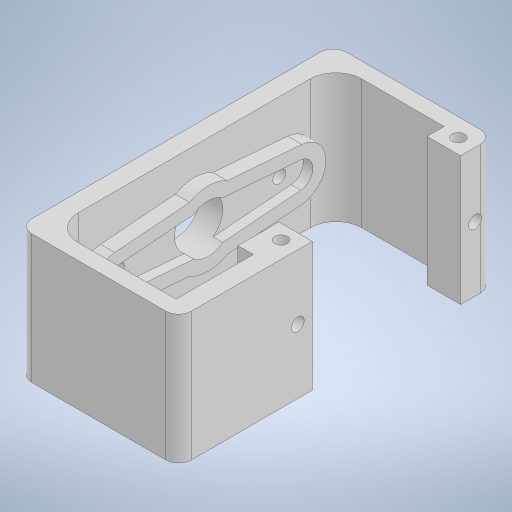
# Autodesk Inventor part: joint4
Saved by Autodesk Inventor 2023 (Build 270158000, 158)
## iProperties
Created: 2023-04-30
Part Number: joint4
Material: 一般
Document SubType Name: Modeling
Designer: taka2
Density: 1 g/cm^3
Appearance: 既定
Author: taka2
Autodesk Inventor part; units mm, degrees
ref_plane "YZ Plane" through (0, 0, 0) normal (1, 0, 0) x (0, 1, 0)
ref_plane "XZ Plane" through (0, 0, 0) normal (0, 1, 0) x (-1, 0, 0)
ref_plane "XY Plane" through (0, 0, 0) normal (0, 0, 1) x (1, 0, 0)
sketch "スケッチ1" plane through (0, 0, 0) normal (0, 1, 0) x (-1, 0, 0)
  line L0 (34.0614, 0) -> (-44.6235, 0)
  line L1 (0, 24.4) -> (0, -24.4)
  line L2 (0, -24.4) -> (-24.8, -24.4)
  line L3 (-24.8, -24.4) -> (-24.8, -22)
  line L4 (-24.8, -22) -> (-2.8, -22)
  line L5 (-2.8, -22) -> (-2.8, 22)
  line L6 (-2.8, 22) -> (-24.8, 22)
  line L7 (-24.8, 22) -> (-24.8, 24.4)
  line L8 (-24.8, 24.4) -> (0, 24.4)
  point P0 (0, 0)
  dimension "d0" = 2.8
  dimension "d1" = 48.8
  dimension "d2" = 24.4
  dimension "d3" = 2.4
  dimension "d4" = 2.4
  dimension "d5" = 22
  constraints: 18 end point, 4 perpendicular, 3 horizontal, 2 vertical, 1 collinear, 1 midpoint, 1 point on line
  measures "d0" distance between parallel lines of L1 L5
  measures "d1" distance of L1.start L1.end
  measures "d2" distance of L1.start point (0, 0)
  measures "d3" distance between parallel lines of L8 L6
  measures "d4" distance between parallel lines of L4 L2
  measures "d5" distance of L3.end L4.end
extrude "押し出し1" add sketch "スケッチ1" along normal blind 20
sketch "スケッチ2" plane through (2.8, 0, 22) normal (1, 0, 0) x (0, 0, -1)
  line L0 (0, 20) -> (44, 20) projected
  line L1 (22, 20) -> (22, 0)
  line L2 (0, 0) -> (44, 0) projected
  line L3 (-2.4, 0) -> (-2.4, 20) projected
  line L4 (-2.4, 10) -> (46.4, 10)
  line L5 (46.4, 0) -> (46.4, 20) projected
  circle A0 centre (22, 10) radius 3.75
  arc A1 (7.6386, 12.0436) -> (7.6386, 7.9564) centre (7.8, 10) ccw
  line L6 (19.75, 13) -> (7.6386, 12.0436)
  line L7 (19.75, 7) -> (7.6386, 7.9564)
  circle A2 centre (9.5, 10) radius 1
  arc A3 (36.3614, 7.9564) -> (36.3614, 12.0436) centre (36.2, 10) ccw
  line L8 (24.25, 13) -> (36.3614, 12.0436)
  line L9 (24.25, 7) -> (36.3614, 7.9564)
  circle A4 centre (34.5, 10) radius 1
  line L10 (19.0799, 14.9533) -> (7.4812, 14.0374)
  arc A5 (7.4812, 14.0374) -> (7.4812, 5.9626) centre (7.8, 10) ccw
  line L11 (7.4812, 5.9626) -> (19.0799, 5.0467)
  circle A6 centre (22, 10) radius 5.75
  line L12 (24.9201, 14.9533) -> (36.5188, 14.0374)
  arc A7 (36.5188, 5.9626) -> (36.5188, 14.0374) centre (36.2, 10) ccw
  line L13 (36.5188, 5.9626) -> (24.9201, 5.0467)
  point P0 (18.25, 10)
  point P1 (22, 6.25)
  point P2 (24.25, 13)
  point P3 (24.25, 7)
  point P4 (19.75, 7)
  point P5 (27.0332, 12.7802)
  point P6 (27.0332, 7.2198)
  point P7 (16.9668, 12.7802)
  point P8 (16.9668, 7.2198)
  dimension "d9" = 7.5
  dimension "d8" = 24.4
  dimension "d10" = 6
  dimension "d11" = 14.2
  dimension "d12" = 2.05
  dimension "d13" = 2
  dimension "d14" = 12.5
  dimension "d34" = 2
  dimension "d35" = 2
  dimension "d36" = 2
  constraints: 20 end point, 12 point on circle, 8 symmetric about line, 7 centre point, 6 midpoint, 3 tangent, 2 point on line, 1 vertical, 7 other
  measures "d8" distance from line of L1.start L3
  measures "d10" distance of L7.start L6.start
  measures "d11" distance of A6.centre A1.centre
  measures "d12" radius of A1
  measures "d13" diameter of A2
  measures "d14" distance of A6.centre A2.centre
  measures "d34" distance between parallel lines of L6 L10
  measures "d36" distance between parallel lines of L8 L12
extrude "押し出し2" cut sketch "スケッチ2" against normal through all contours A0 L4 L1 | L1 L4 A0 | L4 A0 L1 | L1 A0 L4 | A4 L4 | L4 A4 | A2 L4 | L4 A2
extrude "押し出し6" add sketch "スケッチ2" along normal blind 2.2 contours A6 L8 A0 L1 | L1 A0 L6 A6 | L12 A7 L4 A3 L8 A6 | A6 L6 A1 L4 A5 L10 | A0 L9 A6 L1 | L1 A6 L7 A0 | A7 L13 A6 L9 A3 L4 | L4 A1 L7 A6 L11 A5
extrude "押し出し3" add sketch "スケッチ2" along normal blind 0.7 contours L8 A6 L4 A0 | A0 L4 A6 L6 | L8 A3 L4 A4 A6 | A6 L4 A2 A1 L6 | A0 L7 A6 L4 | L4 A6 L9 A0 | L4 A4 A3 L9 A6 | A6 L7 A1 L4 A2
sketch "スケッチ3" plane through (24.8, 0, -22) normal (1, 0, 0) x (0, 0, -1)
  line L0 (-46.4, 0) -> (-46.4, 20) projected
  line L1 (2.4, 0) -> (-46.4, 0) projected
  line L2 (-46.4, 20) -> (-25.65, 20)
  line L3 (-25.65, 20) -> (-25.65, 0)
  line L4 (-25.65, 0) -> (-46.4, 0)
  line L5 (-46.4, 0) -> (-46.4, 20)
  line L6 (2.4, 20) -> (-46.4, 20) projected
  line L7 (2.4, 20) -> (-2.65, 20)
  line L8 (-2.65, 20) -> (-2.65, 0)
  line L9 (-2.65, 0) -> (2.4, 0)
  line L10 (2.4, 0) -> (2.4, 20)
  line L11 (-46.4, 10) -> (2.4, 10)
  line L12 (-19.4, 20) -> (-19.4, 0)
  circle A0 centre (-27.9, 10) radius 1
  circle A1 centre (-0.4, 10) radius 1
  point P0 (-22, 0)
  point P1 (-2.65, 20)
  point P2 (-2.65, 0)
  point P3 (2.4, 0)
  dimension "d19" = 27
  dimension "d20" = 6.25
  dimension "d21" = 16.75
  dimension "d22" = 2.25
  dimension "d23" = 2.25
  dimension "d24" = 2
  constraints: 20 end point, 6 point on line, 4 parallel, 2 centre point, 2 horizontal, 2 midpoint, 2 perpendicular, 1 equal radius, 1 vertical
  measures "d19" distance of L12.start L0.end
  measures "d20" distance of L2.end L12.start
  measures "d21" distance of L7.end L12.start
  measures "d22" distance from line of L3 A0.centre
  measures "d23" distance from line of L8 A1.centre
  measures "d24" diameter of A0
extrude "押し出し4" add sketch "スケッチ3" against normal blind 5.2 contours L0 L11 A0 L3 L1 | L0 L2 L3 L11 A0 | L8 L11 A1 L10 L1 | L8 L6 L10 L11 A1
extrude "押し出し8" cut sketch "スケッチ3" against normal blind 5 contours A1 L11 | L11 A1
sketch "スケッチ4" plane through (0, 20, 0) normal (0, 1, 0) x (1, 0, 0)
  line L0 (22.2, 20.9661) -> (22.2, -25.0757)
  line L1 (19.6, -22) -> (19.6, -3.65) projected
  circle A0 centre (22.2, -5.9) radius 1
  circle A1 centre (22.2, 21.6) radius 1
  line L2 (24.8, -3.65) -> (19.6, -3.65) projected
  line L3 (24.8, 19.35) -> (19.6, 19.35) projected
  line L4 (24.8, -24.4) -> (24.8, -3.65) projected
  point P0 (0, 0)
  point P1 (24.8, -24)
  dimension "d28" = 2.6
  dimension "d29" = 2.25
  dimension "d30" = 2
  dimension "d31" = 2.25
  constraints: 2 centre point, 2 end point, 2 point on line, 1 equal radius, 1 vertical
  measures "d28" distance between parallel lines of L0 L1
  measures "d29" distance from line of L2 A0.centre
  measures "d30" diameter of A0
  measures "d31" distance from line of L3 A1.centre
extrude "押し出し5" cut sketch "スケッチ4" against normal blind 7
sketch "スケッチ5" plane through (0, 20, 0) normal (0, 1, 0) x (1, 0, 0)
  line L0 (19.6, -22) -> (2.8, -22) projected
  line L1 (19.6, -22) -> (22, -22)
  line L2 (22, -22) -> (22, -10)
  line L3 (22, -10) -> (19.6, -10)
  line L4 (19.6, -22) -> (19.6, -3.65) projected
  line L5 (24.8, -24.4) -> (24.8, -3.65) projected
  point P0 (0, 0)
  dimension "d39" = 2.8
  dimension "d40" = 12
  constraints: 6 end point, 2 perpendicular, 1 horizontal, 1 point on line
  measures "d39" distance between parallel lines of L5 L2
  measures "d40" distance between parallel lines of L1 L3
extrude "押し出し7" cut sketch "スケッチ5" against normal through all
fillet "フィレット2" radius 2 2 edges at (0, 10, 24.4) (0, 10, -24.4)
fillet "フィレット4" radius 2 2 edges at (24.8, 10, 24.4) (24.8, 10, -24.4)
fillet "フィレット5" radius 4 1 edges at (2.8, 10, -22)
fillet "フィレット6" radius 4 1 edges at (2.8, 10, 22)
